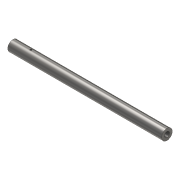
# Autodesk Inventor part: Eje_Base
Saved by Autodesk Inventor 2022 (Build 260153000, 153)
## iProperties
Created: 2019-06-25
Part Number: Eje_Base
Material: Acero, carbono
Document SubType Name: Modeling
Designer: Cristiano
Density: 7.85 g/cm^3
Appearance: Semipulido
Author: Cristiano
Autodesk Inventor part; units mm, degrees
ref_plane "YZ Plane" through (0, 0, 0) normal (1, 0, 0) x (0, 1, 0)
ref_plane "XZ Plane" through (0, 0, 0) normal (0, 1, 0) x (-1, 0, 0)
ref_plane "XY Plane" through (0, 0, 0) normal (0, 0, 1) x (1, 0, 0)
sketch "Boceto1" plane through (0, 0, 0) normal (0, 0, 1) x (1, 0, 0)
  line L0 (0, 0) -> (290, 0)
  line L1 (290, 0) -> (290, 10)
  line L2 (0, 10) -> (0, 0)
  line L3 (290, 10) -> (0, 10)
  dimension "d0" = 10
  dimension "d1" = 290
  constraints: 8 end point, 2 parallel, 1 horizontal, 1 perpendicular
  measures "d0" distance of L2.start L0.start
  measures "d1" distance of L0.start L0.end
revolve "Revolución1" add sketch "Boceto1" angle 360 about axis through (0, 0, 0) along (1, 0, 0)
sketch "Boceto3" plane through (290, 0, 0) normal (1, 0, 0) x (0, 0, -1)
  circle A0 centre (0, 0) radius 5
  dimension "d10" = 10
  constraints: 1 centre point, 1 coincident
  measures "d10" diameter of A0
extrude "Extrusión2" cut sketch "Boceto3" against normal blind 15
thread "Rosca1" size "M10x1.5" class "6H" standard "ANSI Metric M Profile" full length
sketch "Sketch4" plane through (0, 0, 0) normal (0, 0, 1) x (1, 0, 0)
  circle A0 centre (33.75, 0) radius 1.5
  line L0 (0, -10) -> (0, 10) projected
  point P0 (0, 0)
  dimension "d15" = 3
  dimension "d16" = 33.75
  constraints: 1 centre point
  measures "d15" diameter of A0
  measures "d16" distance from line of L0 A0.centre
extrude "Extrusion3" cut sketch "Sketch4" along normal blind 33.75
thread "Thread2" size "M3x0.5" class "6H" standard "ANSI Metric M Profile" full length
equation "\"d17\" = d16"
